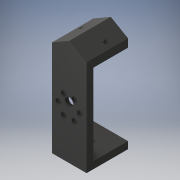
# Autodesk Inventor part: BO12
Saved by Autodesk Inventor 2017 (Build 210142000, 142)
## iProperties
Created: 2018-10-22
Part Number: BO12
Material: ABS Plastic
Document SubType Name: Modeling
Designer: Dell
Density: 1.06 g/cm^3
Appearance: Smooth - Black
Author: Dell
Autodesk Inventor part; units mm, degrees
ref_plane "YZ Plane" through (0, 0, 0) normal (1, 0, 0) x (0, 1, 0)
ref_plane "XZ Plane" through (0, 0, 0) normal (0, 1, 0) x (-1, 0, 0)
ref_plane "XY Plane" through (0, 0, 0) normal (0, 0, 1) x (1, 0, 0)
sketch "Sketch1" plane through (0, 0, 0) normal (0, 0, 1) x (1, 0, 0)
  line L0 (0, 0) -> (0, 152.8559)
  line L1 (0, 152.8559) -> (-25, 138.4222)
  line L2 (-25, 138.4222) -> (-25, 0)
  line L3 (-25, 0) -> (25, 0)
  line L4 (25, 0) -> (25, 138.4222)
  line L5 (25, 138.4222) -> (0, 152.8559)
  dimension "d0" = 152.8559
  dimension "d1" = 60
  dimension "d2" = 60
  dimension "d3" = 50
  constraints: 12 end point, 2 perpendicular, 2 vertical, 1 midpoint
  measures "d0" distance of L0.start L0.end
  measures "d1" angle of L0 L5
  measures "d2" angle of L1 L0
  measures "d3" distance between parallel lines of L4 L2
extrude "Extrusion1" add sketch "Sketch1" along normal blind 10
sketch "Sketch2" plane through (0, 0, 0) normal (0, 0, -1) x (-1, 0, 0)
  line L0 (0, 152.8559) -> (25, 138.4222) projected
  line L1 (-25, 138.4222) -> (0, 152.8559) projected
  line L2 (25, 0) -> (-25, 0) projected
  line L3 (-25, 0) -> (25, 0)
  line L4 (25, 0) -> (25, 10)
  line L5 (25, 10) -> (-25, 10)
  line L6 (-25, 10) -> (-25, 0)
  line L7 (25, 138.4222) -> (25, 0) construction
  line L8 (-25, 0) -> (-25, 138.4222) construction
  line L9 (-25, 126.8751) -> (0, 141.3089)
  line L10 (0, 141.3089) -> (25, 126.8751)
  line L11 (25, 138.4222) -> (25, 0) projected
  line L12 (-25, 126.8751) -> (-25, 138.4222)
  line L13 (0, 152.8559) -> (25, 138.4222) projected
  line L14 (25, 126.8751) -> (25, 138.4222)
  point P0 (0, 0)
  dimension "d6" = 10
  dimension "d7" = 10
  constraints: 16 end point, 4 parallel, 3 point on line, 1 collinear, 1 horizontal, 1 perpendicular, 1 vertical, 1 vertical alignment
  measures "d6" distance between parallel lines of L2 L5
  measures "d7" distance between parallel lines of L1 L9
extrude "Extrusion2" add sketch "Sketch2" along normal blind 50
sketch "Sketch3" plane through (0, 141.3089, -50) normal (-0.5, -0.8660254, 0) x (0.8660254, -0.5, 0)
  circle A0 centre (14.4338, 25) radius 2.5
  line L0 (28.8675, 50) -> (28.8675, 0) projected
  line L1 (28.8675, 0) -> (0, 0) projected
  point P0 (70.6545, 50)
  point P1 (14.4338, 0)
  point P2 (28.8675, 25)
  dimension "d10" = 5
  constraints: 2 midpoint, 1 centre point, 1 horizontal alignment, 1 vertical alignment
  measures "d10" diameter of A0
extrude "Extrusion3" cut sketch "Sketch3" against normal through all
sketch "Sketch4" plane through (-25, 126.8751, -50) normal (0.5, -0.8660254, 0) x (0.8660254, 0.5, 0)
  line L0 (0, 50) -> (0, 0) projected
  line L1 (28.8675, 0) -> (0, 0) projected
  circle A0 centre (14.4338, 25) radius 2.5
  point P0 (-41.7869, 50)
  point P1 (14.4338, 0)
  point P2 (0, 25)
  dimension "d13" = 5
  constraints: 2 midpoint, 1 centre point, 1 horizontal alignment, 1 vertical alignment
  measures "d13" diameter of A0
extrude "Extrusion4" cut sketch "Sketch4" against normal through all
sketch "Sketch5" plane through (-25, 10, 0) normal (0, 1, 0) x (1, 0, 0)
  line L0 (0, 0) -> (0, 50) projected
  line L1 (0, 50) -> (50, 50) projected
  circle A0 centre (25, 25) radius 2.5
  point P0 (25, 0)
  point P1 (25, 50)
  point P2 (0, 25)
  dimension "d16" = 5
  constraints: 2 midpoint, 1 centre point, 1 horizontal alignment, 1 vertical alignment
  measures "d16" diameter of A0
extrude "Extrusion5" cut sketch "Sketch5" against normal through all
sketch "Sketch6" plane through (0, 0, 10) normal (0, 0, 1) x (1, 0, 0)
  circle A0 centre (0, 76.428) radius 6
  line L0 (-25, 138.4222) -> (0, 152.8559) construction
  line L1 (0, 152.8559) -> (0, 0) construction
  circle A1 centre (0, 69.428) radius 1.5 construction
  circle A2 centre (15.5, 69.428) radius 1.5
  circle A3 centre (7.75, 82.8513) radius 1.5
  circle A4 centre (-7.75, 82.8513) radius 1.5
  circle A5 centre (-15.5, 69.428) radius 1.5
  circle A6 centre (-7.75, 56.0046) radius 1.5
  circle A7 centre (7.75, 56.0046) radius 1.5
  point P0 (0, 76.428)
  dimension "d19" = 12
  dimension "d22" = 3
  dimension "d23" = 7
  dimension "d24" = 3
  dimension "d25" = 15.5
  dimension "d28" = 360
  constraints: 8 centre point, 2 end point, 1 coincident, 1 horizontal alignment, 1 midpoint, 1 point on line, 1 vertical, 13 other
  measures "d19" diameter of A0
  measures "d22" diameter of A1
  measures "d23" distance of A0.centre A1.centre
  measures "d24" diameter of A2
  measures "d25" distance of A1.centre A2.centre
extrude "Extrusion6" cut sketch "Sketch6" against normal through all
sketch "Sketch7" plane through (0, 0, 0) normal (0, 0, -1) x (-1, 0, 0)
  circle A0 centre (-7.75, 56.0046) radius 1.5 projected
  circle A1 centre (15.5, 69.428) radius 1.5 projected
  circle A2 centre (-7.75, 82.8513) radius 1.5 projected
  circle A3 centre (-15.5, 69.428) radius 1.5 projected
  circle A4 centre (7.75, 82.8513) radius 1.5 projected
  circle A5 centre (7.75, 56.0046) radius 1.5 projected
  circle A6 centre (0, 76.428) radius 6 projected
  line L0 (-25, 10) -> (25, 10) projected
  line L1 (25, 126.8751) -> (25, 10) projected
  line L2 (25, 126.8751) -> (0, 141.3089) projected
  line L3 (0, 141.3089) -> (-25, 126.8751) projected
  line L4 (-25, 10) -> (-25, 126.8751) projected
  circle A7 centre (0, 69.428) radius 20
  point P0 (0, 0)
  dimension "d32" = 40
  constraints: 1 centre point, 1 horizontal alignment, 1 vertical alignment
  measures "d32" diameter of A7
extrude "Extrusion7" cut sketch "Sketch7" against normal blind 5 contours A0 | A1 | A2 | A3 | A4 | A5 | A6 | A7
sketch "Sketch8" plane through (0, 0, 10) normal (0, 0, 1) x (1, 0, 0)
  circle A0 centre (15.5, 69.428) radius 1.5 projected
  circle A1 centre (0, 69.428) radius 1.5
  line L0 (-25, 0) -> (25, 0) projected
  circle A2 centre (15.5, 69.428) radius 4
  circle A3 centre (7.75, 82.8513) radius 4
  circle A4 centre (-7.75, 82.8513) radius 4
  circle A5 centre (-15.5, 69.428) radius 4
  circle A6 centre (-7.75, 56.0046) radius 4
  circle A7 centre (7.75, 56.0046) radius 4
  point P0 (0, 0)
  point P1 (0, 0)
  dimension "d35" = 3
  dimension "d36" = 8
  dimension "d39" = 360
  constraints: 7 centre point, 1 coincident, 1 horizontal alignment, 1 midpoint, 1 vertical alignment, 13 other
  measures "d35" diameter of A1
  measures "d36" diameter of A2
extrude "Extrusion8" cut sketch "Sketch8" against normal blind 3 contours A0 | A2 | A3 | A4 | A5 | A6 | A7
body "Solid1"
